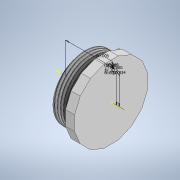
# Autodesk Inventor part: 1aThreadsV04-1_3-4x12-externalTest
Saved by Autodesk Inventor 2021.1 (Build 251245010, 245A)
## iProperties
Created: 2020-10-17
Part Number: 1aThreadsV04-1_3-4x12-externalTest
Material: Generic
Document SubType Name: Modeling
Designer: robst
Density: 1 g/cm^3
Appearance: Default
Author: robst
Autodesk Inventor part; units mm, degrees
ref_plane "XZ Plane" through (0, 0, 0) normal (0, 1, 0) x (-1, 0, 0)
ref_plane "XY Plane" through (0, 0, 0) normal (0, 0, 1) x (1, 0, 0)
sketch "ExternalTheadSketch" plane through (0, 0, 0) normal (0, 0, 1) x (1, 0, 0)
  line L0 (25.4, 22.0929) -> (29.6333, 22.0929) construction
  line L1 (29.6333, 22.0929) -> (29.6333, 20.7759) construction
  line L2 (29.6333, 20.7759) -> (25.4, 20.7759) construction
  line L3 (25.4, 20.7759) -> (25.4, 22.0929) construction
  line L4 (26.7271, 21.9377) -> (27.3385, 20.8788)
  line L5 (27.6948, 20.8788) -> (28.3062, 21.9377)
  arc A0 (27.3385, 20.8788) -> (27.6948, 20.8788) centre (27.5167, 20.9817) ccw
  arc A1 (26.7271, 21.9377) -> (26.4583, 22.0929) centre (26.4583, 21.7826) ccw
  arc A2 (28.575, 22.0929) -> (28.3062, 21.9377) centre (28.575, 21.7826) ccw
  line L6 (26.4583, 22.0929) -> (28.575, 22.0929)
  point P0 (0, 0)
  dimension "d44" = 25.4
  dimension "d45" = 22.0929
  dimension "d46" = 20.7759
  dimension "d47" = 60
  dimension "d48" = 0.2057
  dimension "d54" = 1.0583
  dimension "d55" = 2.1167
  dimension "d56" = 4.2333
  constraints: 14 end point, 7 tangent, 6 point on circle, 3 centre point, 2 parallel, 1 equal radius, 1 horizontal, 1 perpendicular
  measures "d44" distance from line of L3 point (0, 0)
  measures "d45" distance from line of point (0, 0) L0
  measures "d46" distance from line of point (0, 0) L2
  measures "d47" angle of L5 L4
  measures "d48" radius of A0
  measures "d54" distance from line of A1.centre L3
  measures "d55" distance of A2.centre A1.centre
  measures "d56" distance between parallel lines of L1 L3
sketch "InternalThreadSketch" plane through (0, 0, 0) normal (0, 0, 1) x (1, 0, 0)
  line L0 (32.0383, 21.1938) -> (32.6879, 22.319)
  line L1 (32.8859, 22.319) -> (33.5356, 21.1938)
  arc A0 (32.8859, 22.319) -> (32.6879, 22.319) centre (32.7869, 22.2618) ccw
  line L2 (32.0383, 21.1938) -> (31.4617, 21.1938)
  line L3 (33.5356, 21.1938) -> (34.1121, 21.1938)
  line L4 (-6.8224, 0) -> (40.9346, 0) projected
  line L5 (31.75, 21.1938) -> (33.8667, 21.1938) construction
  line L6 (33.8667, 21.1938) -> (33.8667, 22.3761) construction
  line L7 (33.8667, 22.3761) -> (31.75, 22.3761) construction
  line L8 (31.75, 22.3761) -> (31.75, 21.1938) construction
  line L9 (32.0383, 21.1938) -> (33.5356, 21.1938)
  point P0 (0, 0)
  dimension "d71" = 60
  dimension "d72" = 0.1143
  dimension "d73" = 0.5766
  dimension "d75" = 22.3761
  dimension "d76" = 21.1938
  dimension "d77" = 120
  dimension "d78" = 31.75
  dimension "d79" = 2.1167
  constraints: 18 end point, 3 collinear, 3 horizontal, 3 tangent, 2 parallel, 2 point on circle, 1 centre point, 1 midpoint, 1 perpendicular
  measures "d71" angle of L1 L0
  measures "d72" radius of A0
  measures "d73" distance of L0.start L2.end
  measures "d76" distance between parallel lines of L3 L4
  measures "d77" angle of L0 L2
  measures "d78" distance from line of L8 point (0, 0)
  measures "d79" distance between parallel lines of L6 L8
ref_plane "Work Plane1" through (25.4, 0, 0) normal (1, 0, 0) x (0, 1, 0)
sketch "Sketch3" plane through (25.4, 0, 0) normal (1, 0, 0) x (0, 1, 0)
  circle A0 centre (0, 0) radius 22.0929
  dimension "d81" = 44.1858
  constraints: 1 centre point, 1 coincident
  measures "d81" diameter of A0
extrude "Extrusion1" add sketch "Sketch3" against normal blind 12.7
coil "Coil1" sketch "ExternalTheadSketch" operation cut axis through (-10, 0, 0) along (-1, 0, 0) pitch 2.1167 turns 8 hand right
sketch "Sketch4" plane through (25.4, 0, 0) normal (1, 0, 0) x (0, 1, 0)
  line L0 (5.0524, -25.4) -> (-5.0524, -25.4)
  line L1 (-5.0524, -25.4) -> (-14.3879, -21.5331)
  line L2 (-14.3879, -21.5331) -> (-21.5331, -14.3879)
  line L3 (-21.5331, -14.3879) -> (-25.4, -5.0524)
  line L4 (-25.4, -5.0524) -> (-25.4, 5.0524)
  line L5 (-25.4, 5.0524) -> (-21.5331, 14.3879)
  line L6 (-21.5331, 14.3879) -> (-14.3879, 21.5331)
  line L7 (-14.3879, 21.5331) -> (-5.0524, 25.4)
  line L8 (-5.0524, 25.4) -> (5.0524, 25.4)
  line L9 (5.0524, 25.4) -> (14.3879, 21.5331)
  line L10 (14.3879, 21.5331) -> (21.5331, 14.3879)
  line L11 (21.5331, 14.3879) -> (25.4, 5.0524)
  line L12 (25.4, 5.0524) -> (25.4, -5.0524)
  line L13 (25.4, -5.0524) -> (21.5331, -14.3879)
  line L14 (21.5331, -14.3879) -> (14.3879, -21.5331)
  line L15 (14.3879, -21.5331) -> (5.0524, -25.4)
  point P0 (0, 0)
  point P1 (0, 0)
  dimension "d93" = 50.8
  constraints: 32 end point, 1 coincident, 1 horizontal, 33 other
  measures "d93" distance between parallel lines of L8 L0
extrude "Extrusion2" add sketch "Sketch4" along normal blind 6.35
sketch "Sketch5" plane through (12.7, 0, 0) normal (-1, 0, 0) x (0, 0, 1)
  circle A0 centre (0, 0) radius 19.05
  dimension "d96" = 38.1
  constraints: 1 centre point, 1 coincident
  measures "d96" diameter of A0
extrude "Extrusion3" cut sketch "Sketch5" against normal blind 12.7
equation "\"d45\" = a1MajorRadius"
equation "\"d46\" = a1MinorRadius"
equation "\"d47\" = threadAngle"
equation "\"d48\" = a1RootRadius"
equation "\"d54\" = 0.5 * pitch"
equation "\"d55\" = pitch"
equation "\"d56\" = 2 * pitch"
equation "\"d71\" = threadAngle"
equation "\"d72\" = b1RootRadius"
equation "\"d73\" = b1CrestFlat"
equation "\"d75\" = b1MajorRadius"
equation "\"d76\" = b1MinorRadius"
equation "\"d79\" = pitch"
equation "\"d81\" = a1MajorDiameter"
equation "\"d85\" = pitch"
equation "\"threadAngle\" = 60deg"
equation "\"a1MajorDiameter\" = 44.18584"
equation "\"a1MajorRadius\" = 0.5 * a1MajorDiameter"
equation "\"a1MinorDiameter\" = 41.55186"
equation "\"a1MinorRadius\" = 0.5 * a1MinorDiameter"
equation "\"a1RootRadius\" = 0.20574"
equation "\"a1CrestRadiusMax\" = 0.2286"
equation "\"a1ThreadDepth\" = 1.34366"
equation "\"b1MajorDiameter\" = 44.75226"
equation "\"b1MajorRadius\" = 0.5 * b1MajorDiameter"
equation "\"b1MinorDiameter\" = 42.38752"
equation "\"b1RootRadius\" = 0.1143"
equation "\"b1MinorRadius\" = 0.5 * b1MinorDiameter"
equation "\"b1ThreadDepth\" = 1.1811"
equation "\"b1CrestFlat\" = 0.57658"
equation "\"pitch\" = 2.116667"
body "Solid1"
